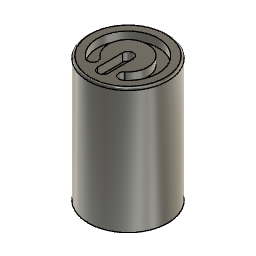
Button v8 (Autodesk Fusion 360 design; units mm, degrees)
Autodesk Fusion 360 part; units mm, degrees
sketch "Skizze1" plane through (0, 0, 0) normal (0, 0, 1) x (1, 0, 0)
  circle A0 centre (0, 0) radius 3.9
  dimension "d1" = 7.8
  constraint coincident A0.centre origin
  measures "d1" diameter of A0
extrude "Extrusion1" add sketch "Skizze1" along normal blind 12
sketch "Skizze2" plane through (0, 0, 12) normal (0, 0, 1) x (-1, 0, 0)
  circle A0 centre (0, 0) radius 3.9
  line L0 (1.05, 1.3) -> (-1.05, 1.3)
  line L1 (-1.05, 1.3) -> (-1.05, -1.3)
  line L2 (-1.05, -1.3) -> (1.05, -1.3)
  line L3 (1.05, -1.3) -> (1.05, 1.3)
  line L4 (1.05, 1.3) -> (-1.05, -1.3) construction
  line L5 (-1.05, 1.3) -> (1.05, -1.3) construction
  dimension "d4" = 2.1
  dimension "d5" = 2.6
  constraint horizontal L0
  constraint perpendicular L0 L1
  constraint parallel L0 L2
  constraint parallel L1 L3
  constraint coincident L4 A0.centre
  constraint coincident L5 A0.centre
  constraint coincident A0.centre origin
  measures "d4" distance of L1.end L2.end
  measures "d5" distance of L0.end L1.end
extrude "Extrusion2" cut sketch "Skizze2" against normal blind 2.5 contours L0 L1 L2 L3
sketch "Skizze3" plane through (0, 0, 0) normal (0, 0, -1) x (1, 0, 0)
  circle A0 centre (0, 0) radius 3.9
  circle A1 centre (0, 0) radius 2.9
  circle A2 centre (0, 0) radius 1.9
  line L0 (0, 3.9) -> (0, 2.9)
  circle A3 centre (0, 2.9) radius 0.5
  line L1 (0, 2.9) -> (0, 0.9)
  circle A4 centre (0, 0.9) radius 0.5
  line L2 (-0.5, 0.9) -> (0.5, 0.9)
  line L3 (0.5, 0.9) -> (0.5, 2.9)
  line L4 (0.5, 2.9) -> (-0.5, 2.9)
  line L5 (-0.5, 2.9) -> (-0.5, 0.9)
  line L6 (-0.5, 0.9) -> (0.5, 2.9) construction
  line L7 (0.5, 0.9) -> (-0.5, 2.9) construction
  circle A5 centre (-1.5, 1.8735) radius 0.5
  line L8 (1, 0.9) -> (-1, 0.9)
  line L9 (-1, 0.9) -> (-1, 2.9)
  line L10 (-1, 2.9) -> (1, 2.9)
  line L11 (1, 2.9) -> (1, 0.9)
  line L12 (1, 0.9) -> (-1, 2.9) construction
  line L13 (-1, 0.9) -> (1, 2.9) construction
  circle A6 centre (1.5, 1.8735) radius 0.5
  point P0 (0, 1.9)
  point P1 (0, 1.9)
  dimension "d8" = 5.8
  dimension "d9" = 3.8
  dimension "d10" = 1
  dimension "d11" = 2
  dimension "d12" = 2
  dimension "d13" = 1
  constraint coincident A0.centre A1.centre
  constraint coincident A0 L0.start
  constraint coincident A1 L0.end
  constraint vertical L0
  constraint coincident L0.end A3.centre
  constraint parallel L0 L1
  constraint coincident L1.end A4.centre
  constraint horizontal L2
  constraint perpendicular L2 L3
  constraint parallel L2 L4
  constraint parallel L3 L5
  constraint coincident L6 P1
  constraint coincident L7 P1
  constraint coincident A4 L2.start
  constraint midpoint L1 P1
  constraint horizontal L8
  constraint perpendicular L8 L9
  constraint parallel L8 L10
  constraint parallel L9 L11
  constraint coincident L12 P1
  constraint coincident L13 P1
  constraint coincident P1 P0
  constraint tangent A5 L9
  constraint tangent A1 A5
  constraint tangent L11 A6
  constraint tangent A1 A6
  measures "d8" diameter of A1
  measures "d9" diameter of A2
  measures "d10" diameter of A5
  measures "d11" distance of L9.end L10.end
  measures "d12" distance of L8.end L9.end
  measures "d13" diameter of A6
extrude "Extrusion3" cut sketch "Skizze3" against normal blind 0.5 contours A1 A2 A5 A6 | A6 | A5 | A1 A3 L1 | A2 A3 L1 L3 | A1 A3 L3 L4 L10 | A1 A3 L4 L5 L10 | A1 A3 L1 | A2 A3 L1 L5 | L0 A3 L4 L10 | L0 A3 L4 L10 | A2 L1 A4 L3 | A2 L1 A4 L5 | L1 A4 L2 L8 | A4 L2 L8 | L1 A4 L2 L8
fillet "Abrundung1" radius 0.25 1 edges at (-3.6361, -1.4103, 0)
extrude "Extrusion4" add 1 faces at (0.35, -0.4333, 9.5) along direction (0, 0, 1) blind 2.5
sketch "Skizze4" plane through (0, 0, 12) normal (0, 0, 1) x (-1, 0, 0)
  circle A0 centre (0, 0) radius 3.9
  line L0 (1.3, 1.05) -> (-1.3, 1.05)
  line L1 (-1.3, 1.05) -> (-1.3, -1.05)
  line L2 (-1.3, -1.05) -> (1.3, -1.05)
  line L3 (1.3, -1.05) -> (1.3, 1.05)
  line L4 (1.3, 1.05) -> (-1.3, -1.05) construction
  line L5 (-1.3, 1.05) -> (1.3, -1.05) construction
  dimension "d20" = 2.6
  dimension "d21" = 2.1
  constraint horizontal L0
  constraint perpendicular L0 L1
  constraint parallel L0 L2
  constraint parallel L1 L3
  constraint coincident L4 A0.centre
  constraint coincident L5 A0.centre
  constraint coincident A0.centre origin
  measures "d20" distance of L1.end L2.end
  measures "d21" distance of L0.end L1.end
extrude "Extrusion5" cut sketch "Skizze4" against normal blind 2.5 contours L0 L1 L2 L3
move_body "Verschieben1" bodies 1 to x (-1, 0, 0) y (0, 1, 0) z (0, 0, -1) at (0, 0, 12.25)
delete_face "Fläche löschen1" 1 faces at (1.2377, 3.6839, 12.0818)
sketch "Skizze5" plane through (0, 0, 12.25) normal (0, 0, 1) x (-1, 0, 0)
  circle A0 centre (0, 0) radius 3.9
  line L0 (-0.5, 0.9) -> (-0.5, 2.8566)
  arc A1 (-0.4981, 2.8569) -> (-0.5, 2.8566) centre (0, 0) ccw
  arc A2 (0.4981, 2.8569) -> (-0.4981, 2.8569) centre (0, 2.9) ccw
  arc A3 (0.5, 2.8566) -> (0.4981, 2.8569) centre (0, 0) ccw
  line L1 (0.5, 2.8566) -> (0.5, 0.9)
  arc A4 (-0.5, 0.9) -> (0.5, 0.9) centre (0, 0.9) ccw
  arc A5 (-1.8125, 2.2638) -> (1.8125, 2.2638) centre (0, 0) ccw
  arc A6 (-1.1875, 1.4832) -> (-1.8125, 2.2638) centre (-1.5, 1.8735) ccw
  arc A7 (-1.1875, 1.4832) -> (1.1875, 1.4832) centre (0, 0) ccw
  arc A8 (1.8125, 2.2638) -> (1.1875, 1.4832) centre (1.5, 1.8735) ccw
  circle A9 centre (0, 0) radius 3.8
  dimension "d24" = 7.6
  constraint coincident A0.centre A1.centre
  measures "d24" diameter of A9
extrude "Extrusion6" cut sketch "Skizze5" against normal blind 13 contours A0
extrude "Extrusion7" cut 2 faces at (-0.166, -1.5523, 11.75) (1.378, -1.9871, 11.75) along direction (0, 0, -1) blind 0.3
fillet "Abrundung2" radius 0.2 1 edges at (3.5428, 1.3741, 12.25)
extrude "Extrusion8" add 1 faces at (-0.166, -1.5523, 11.45) along direction (0, 0, 1) blind 0.8
sketch "Skizze6" plane through (0, 0, 12.25) normal (0, 0, 1) x (-1, 0, 0)
  arc A0 (-1.8125, 2.2638) -> (1.8125, 2.2638) centre (0, 0) ccw
  arc A1 (-1.1875, 1.4832) -> (-1.8125, 2.2638) centre (-1.5, 1.8735) ccw
  arc A2 (-1.1875, 1.4832) -> (1.1875, 1.4832) centre (0, 0) ccw
  arc A3 (1.8125, 2.2638) -> (1.1875, 1.4832) centre (1.5, 1.8735) ccw
  circle A4 centre (0, 0) radius 3.6
  line L0 (0, 3.6) -> (0, 2.9)
  line L1 (0, 2.9) -> (0, 2.4)
  circle A5 centre (0, 2.4) radius 0.5
  line L2 (0, 0) -> (0, 0.5)
  circle A6 centre (0, 0.5) radius 0.5
  line L3 (-0.5, 2.4) -> (0.5, 2.4)
  line L4 (0.5, 2.4) -> (0.5, 0.5)
  line L5 (0.5, 0.5) -> (-0.5, 0.5)
  line L6 (-0.5, 0.5) -> (-0.5, 2.4)
  dimension "d33" = 0.7
  dimension "d34" = 0.5
  dimension "d35" = 0.5
  constraint coincident A4 L0.start
  constraint vertical L0
  constraint parallel L0 L1
  constraint coincident L1.end A5.centre
  constraint coincident L0.end A5
  constraint coincident A0.centre A2.centre
  constraint vertical L2
  constraint coincident L2.end A6.centre
  constraint coincident A0.centre A6
  constraint horizontal L3
  constraint vertical L4
  constraint horizontal L5
  constraint vertical L6
  constraint coincident A6 L4.end
  constraint coincident A5 L3.start
  measures "d33" distance of L0.start L0.end
  measures "d34" distance of L0.end L1.end
  measures "d35" distance of A0.centre L2.end
extrude "Extrusion9" cut sketch "Skizze6" against normal blind 0.8 contours L1 A5 L3 | L1 A5 L3 | A5 L3 | A5 A6 L4 L6 | A6 L5 | L2 A6 L5 | L2 A6 L5
sketch "Skizze7" plane through (0, 0, 12.25) normal (0, 0, 1) x (-1, 0, 0)
  line L0 (-0.5, 0.5) -> (-0.5, 2.4)
  arc A0 (0.5, 2.4) -> (-0.5, 2.4) centre (0, 2.4) ccw
  line L1 (0.5, 2.4) -> (0.5, 0.5)
  arc A1 (-0.5, 0.5) -> (0.5, 0.5) centre (0, 0.5) ccw
  arc A2 (-1.8125, 2.2638) -> (1.8125, 2.2638) centre (0, 0) ccw
  arc A3 (-1.1875, 1.4832) -> (-1.8125, 2.2638) centre (-1.5, 1.8735) ccw
  arc A4 (-1.1875, 1.4832) -> (1.1875, 1.4832) centre (0, 0) ccw
  arc A5 (1.8125, 2.2638) -> (1.1875, 1.4832) centre (1.5, 1.8735) ccw
  circle A6 centre (0, 0) radius 3.6
  circle A7 centre (0, 0) radius 0.5
  line L2 (-0.5, 0) -> (-0.5, 0.7)
  line L3 (0.5, 0) -> (0.5, 0.7)
  dimension "d38" = 1
  constraint coincident A2.centre A4.centre
  constraint coincident A7 L2.start
  constraint coincident L0 L2.end
  constraint parallel L0 L2
  constraint coincident A7 L3.start
  constraint coincident L1 L3.end
  measures "d38" diameter of A7
extrude "Extrusion10" cut sketch "Skizze7" against normal blind 0.8 contours A1 A7 L2 | A1 A7 | A1 A7 L3 picked at (0, -0.3324)
